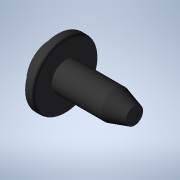
# Autodesk Inventor part: 1301.000_10_(1)
Saved by Autodesk Inventor 2021 (Build 250183000, 183)
## iProperties
Created: 2025-05-02
Part Number: 1301.000_10_(1)
Material: Generic
Catalog Web Link: www.cadenas.de
Description: Schraube KX EB Edelstahl-Schraube KX EB Edelstahl
Vendor: RITTAL
Document SubType Name: Modeling
Designer: psAdmin
Manufacturer: RITTAL
Mass: 0.490021 g
Surface Area: 4.44774 cm^2
Volume: 0.490021 cm^3
Density: 1 g/cm^3
Appearance: PSOLRGB-175-175-175
Category: PARTsolutions
Company: RITTAL
Title: 1301.000_10
Author: Cadenas PARTsolutions
Comments: Schraube KX EB Edelstahl
PSOL_IDENT_0: {$CADENAS_DATA/23d-libs/rittal/schaltschranksys/edelstahl/kleingehause/parts_eb_edel_2_0/schraube_kx
PSOL_IDENT_1: _eb_edel_new.prj},197 {VTYP=3D},{NB=1301.000_10_(1)},{LINA=1301.000_10},{NN=Schraube KX EB Edelstahl
PSOL_IDENT_2: },{DATE=28.04.2025 21:10:48},{GEOMDATE=11.04.2025 11:21:29},{VERSION=},{LINEID=610},{WBVAR=DETAIL},{
PSOL_IDENT_3: WBNUMERIC=DETAIL}  {NB=1301.000_10_(1)},{LINA=1301.000_10},{KT=DUMMY},{BEST=1301.000},{DETAIL=1},{GE
PSOL_IDENT_4: W=3,889},{CNSETIM80=EC000261},{CNSETIM90=EC000261},{CNSECLASS60=27-18-01-01},{CNSECLASS80=27-18-01-0
PSOL_IDENT_5: 1},{UNSPSC=31-26-15-02}
NB: 1301.000_10_(1)
NN: Schraube KX EB Edelstahl
NT: Schraube KX EB Edelstahl
NBSYN: $BEST._10_($DETAIL.)
LINA: 1301.000_10
CATALOG: Rittal
BEST: 1301.000
DETAIL: hoch
GEW: 3,889
CNSETIM80: EC000261
CNSETIM90: EC000261
CNSECLASS60: 27-18-01-01
CNSECLASS80: 27-18-01-01
UNSPSC: 31-26-15-02
SUPPLIER: RITTAL
ARTICLENO: 1301.000_10_(1)
BOMINFO: 1301.000_10
CREATOR: CADENAS GmbH
Autodesk Inventor part; units mm, degrees
sketch "Sketch_1" plane through (0, 0, 0) normal (0, 0, 1) x (1, 0, 0)
  line L0 (12, 0) -> (-3.6, 0)
  line L1 (-3.6, 0) -> (-3.6, 2.6)
  arc A0 (-1.6, 5) -> (-3.6, 2.6) centre (-0.2671, 1.8559) ccw
  line L2 (-1.6, 5) -> (-1.6, 5.45)
  arc A1 (-1.3, 5.75) -> (-1.6, 5.45) centre (-1.3, 5.45) ccw
  line L3 (-1.3, 5.75) -> (-0.425, 5.75)
  arc A2 (0, 5.325) -> (-0.425, 5.75) centre (-0.425, 5.325) ccw
  line L4 (0, 5.325) -> (0, 2.5)
  line L5 (0, 2.5) -> (8.6241, 2.5)
  line L6 (8.6241, 2.5) -> (12, 1.5)
  line L7 (12, 1.5) -> (12, 0)
  line L8 (12, 0) -> (-3.6, 0)
  constraints: 18 end point, 6 point on circle, 3 centre point
revolve "Revolution1" add sketch "Sketch_1" angle 360 about axis through (12, 0, 0) along (1, 0, 0)
ref_plane "SCHRAUBE_XY" through (0, 0, 0) normal (-1, 0, 0) x (0, 0, -1)
ref_plane "SCHRAUBE_YZ" through (0, 0, 0) normal (0, 0, -1) x (0, -1, 0)
ref_plane "SCHRAUBE_ZX" through (0, 0, 0) normal (0, -1, 0) x (-1, 0, 0)
body "Solid1"
